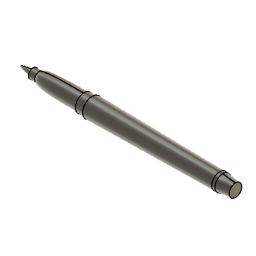
marcador v2 (Autodesk Fusion 360 design; units mm, degrees)
Autodesk Fusion 360 part; units mm, degrees
sketch "Boceto1" plane through (0, 0, 0) normal (0, 1, 0) x (1, 0, 0)
  line L0 (0, 0) -> (0, -4)
  line L1 (0, 0) -> (-10, 0)
  line L2 (-10, 0) -> (-10, -5)
  line L3 (-10, -5) -> (-8, -5)
  line L4 (-8, -5) -> (-8, 0)
  spline S0 degree 5 poles (-8, -5) (-7.6785, -4.9248) (-7.0375, -4.781) (-6.0814, -4.5846) (-4.818, -4.3623) (-3.2588, -4.1548) (-1.985, -4.0466) (-1.0305, -4.006) (-0.3853, -3.9982) (-0.0428, -3.9997) (0, -4) knots 0 0 0 0 0 0 0.1 0.2 0.3 0.4 0.5 0.514308 0.514308 0.514308 0.514308 0.514308 0.514308
  line L5 (-0.7884, -3.9948) -> (0.7884, -4.0052)
  line L6 (-10, 0) -> (-90, 0)
  line L7 (-90, 0) -> (-90, -6)
  line L8 (-90, -6) -> (-10, -5)
  line L9 (-90, 0) -> (-95, 0)
  line L10 (-95, 0) -> (-95, -5.5)
  line L11 (-95, -5.5) -> (-90, -5.5)
  line L12 (-95, 0) -> (-95, -5)
  line L13 (-95, 0) -> (-123, 0)
  line L14 (-123, 0) -> (-123, -3)
  spline S1 degree 5 poles (-95, -5) (-96.2479, -5.0207) (-98.6911, -5.0534) (-102.1981, -5.0763) (-106.553, -5.0536) (-111.4163, -4.929) (-115.6208, -4.6951) (-119.0596, -4.3342) (-121.1676, -3.9138) (-122.2702, -3.5129) (-122.7774, -3.1994) (-122.9773, -3.0213) (-123, -3) knots 0 0 0 0 0 0 0.1 0.2 0.3 0.4 0.5 0.6 0.7 0.713455 0.713455 0.713455 0.713455 0.713455 0.713455
  line L15 (-122.4438, -3.5211) -> (-123.5562, -2.4789)
  line L16 (-123, -3) -> (-127, -3)
  line L17 (-127, -3) -> (-127, 0)
  line L18 (-127, 0) -> (-123, 0)
  line L19 (-127, 0) -> (-135, 0)
  line L20 (-127, 0) -> (-127, -2)
  spline S2 degree 5 poles (-127, -2) (-127.4129, -1.9382) (-128.2169, -1.8145) (-129.3575, -1.6287) (-130.7453, -1.3802) (-132.241, -1.0682) (-133.4686, -0.7548) (-134.3911, -0.4398) (-134.9705, -0.123) (-135.1756, 0.1959) (-135.0021, 0.5168) (-134.574, 0.775) (-134.098, 0.9695) (-133.713, 1.0996) (-133.5035, 1.1647) knots 0 0 0 0 0 0 0.1 0.2 0.3 0.4 0.5 0.6 0.7 0.8 0.9 1 1 1 1 1 1
  dimension "d3" = 4
  dimension "d4" = 10
  dimension "d5" = 5
  dimension "d6" = 2
  dimension "d7" = 80
  dimension "d8" = 6
  dimension "d9" = 5
  dimension "d10" = 5.5
  dimension "d11" = 5
  dimension "d12" = 28
  dimension "d13" = 3
  dimension "d14" = 4
  dimension "d15" = 8
  dimension "d16" = 2
  constraint coincident L0.start L1.start
  constraint vertical L0
  constraint perpendicular L0 L1
  constraint perpendicular L1 L2
  constraint perpendicular L2 L3
  constraint coincident L1 L4.end
  constraint perpendicular L1 L4
  constraint midpoint L0.end L5
  constraint perpendicular L2 L6
  constraint perpendicular L6 L7
  constraint perpendicular L7 L9
  constraint perpendicular L9 L10
  constraint coincident L7 L11.end
  constraint perpendicular L7 L11
  constraint perpendicular L11 L12
  constraint perpendicular L10 L13
  constraint perpendicular L13 L14
  constraint midpoint L14.end L15
  constraint perpendicular L14 L16
  constraint perpendicular L16 L17
  constraint perpendicular L14 L18
  constraint perpendicular L17 L19
  constraint perpendicular L19 L20
  measures "d3" distance of L0.start L0.end
  measures "d4" distance of L0.start L1.end
  measures "d5" distance of L1.end L2.end
  measures "d6" distance of L2.end L3.end
  measures "d7" distance of L1.end L6.end
  measures "d8" distance of L6.end L7.end
  measures "d9" distance of L6.end L9.end
  measures "d10" distance of L9.end L10.end
  measures "d11" distance of L9.end L12.end
  measures "d12" distance of L9.end L13.end
  measures "d13" distance of L13.end L14.end
  measures "d14" distance of L14.end L16.end
  measures "d15" distance of L17.end L19.end
  measures "d16" distance of L17.end L20.end
revolve "Revolución1" add sketch "Boceto1" angle 360 about axis through (-10, 0, 0) along (-1, 0, 0)
